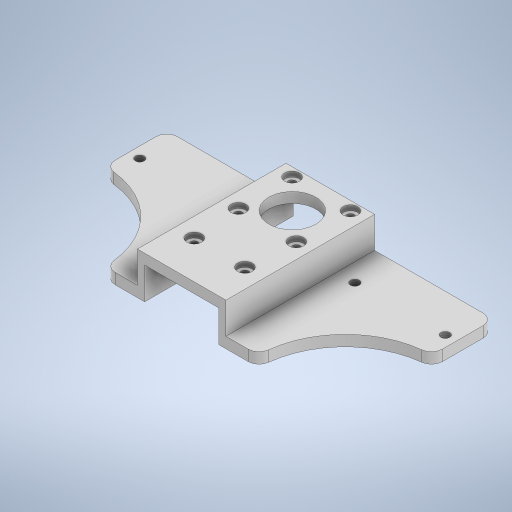
# Autodesk Inventor part: gripper_fixer
Saved by Autodesk Inventor 2024.2 (Build 282272000, 272)
## iProperties
Created: 2023-09-15
Part Number: gripper_fixer
Material: Generic
Document SubType Name: Modeling
Designer: 박동준
Density: 1 g/cm^3
Appearance: Default
Author: 박동준
Autodesk Inventor part; units mm, degrees
ref_plane "YZ Plane" through (0, 0, 0) normal (1, 0, 0) x (0, 1, 0)
ref_plane "XZ Plane" through (0, 0, 0) normal (0, 1, 0) x (-1, 0, 0)
ref_plane "XY Plane" through (0, 0, 0) normal (0, 0, 1) x (1, 0, 0)
sketch "Sketch1" plane through (0, 0, 0) normal (0, 0, 1) x (1, 0, 0)
  line L0 (-12.245, 11.65) -> (-12.245, 3)
  line L1 (-12.245, 3) -> (-45.245, 3)
  line L2 (-45.245, 3) -> (-45.245, 0)
  line L3 (-45.245, 0) -> (-10.245, 0)
  line L4 (-10.245, 0) -> (-10.245, 8.8)
  line L5 (-10.245, 8.8) -> (10.245, 8.8)
  line L6 (10.245, 8.8) -> (10.245, 0)
  line L7 (10.245, 0) -> (45.245, 0)
  line L8 (45.245, 0) -> (45.245, 3)
  line L9 (45.245, 3) -> (12.245, 3)
  line L10 (12.245, 3) -> (12.245, 11.65)
  line L11 (12.245, 11.65) -> (-12.245, 11.65)
  line L12 (-10.245, 0) -> (10.245, 0) construction
  point P0 (0, 0)
  point P1 (0, 11.65)
  point P2 (0, 0)
  point P3 (-12.245, 7.325)
  point P4 (12.245, 7.325)
  dimension "d0" = 20.49
  dimension "d1" = 2.85
  dimension "d3" = 5.8
  dimension "d4" = 3
  dimension "d5" = 3
  dimension "d6" = 35
  dimension "d7" = 35
  dimension "d73" = 33
  dimension "d74" = 33
  constraints: 26 end point, 9 perpendicular, 4 midpoint, 2 point on line, 2 vertical, 1 collinear, 1 horizontal alignment, 1 vertical alignment
  measures "d0" distance between parallel lines of L6 L4
  measures "d1" distance between parallel lines of L11 L5
  measures "d3" distance between parallel lines of L9 L5
  measures "d4" distance of L7.end L8.end
  measures "d5" distance of L1.end L2.end
  measures "d6" distance of L6.end L7.end
  measures "d7" distance of L2.end L3.end
  measures "d73" distance of L0.end L1.end
  measures "d74" distance of L8.end L9.end
extrude "Extrusion1" add sketch "Sketch1" along normal mid plane 41.1
sketch "Sketch8" plane through (12.245, 3, 20.55) normal (0, 1, 0) x (1, 0, 0)
  line L0 (0, 41.1) -> (0, 0)
  line L1 (33, 0) -> (0, 0) projected
  line L2 (33, 41.1) -> (33, 0) projected
  line L3 (0, 41.1) -> (33, 41.1) projected
  line L4 (-57.49, 41.1) -> (-57.49, 0) projected
  line L5 (-24.49, 0) -> (-57.49, 0) projected
  line L6 (-24.49, 0) -> (-24.49, 41.1) projected
  line L7 (-57.49, 41.1) -> (-24.49, 41.1) projected
  line L8 (33, 41.1) -> (33, 0) projected
  circle A0 centre (-11.645, 30.6) radius 6.4 projected
  line L9 (-12.245, 41) -> (-12.245, 0) construction
  point P0 (-12.245, 20.55)
  point P1 (-54.49, 30.65)
  point P2 (-29.49, 30.65)
  point P3 (-57.49, 20.55)
  point P4 (30, 30.65)
  point P5 (5, 30.65)
  dimension "d42" = 3
  dimension "d43" = 25
  dimension "d51" = 10.45
  dimension "d53" = 3
  constraints: 4 end point, 2 symmetric about line, 1 horizontal alignment, 1 midpoint, 1 vertical
  measures "d42" distance from line of L4 point (-54.49, 30.65)
  measures "d43" distance of point (-29.49, 30.65) point (-54.49, 30.65)
  measures "d51" distance from line of point (-29.49, 30.65) L7
  measures "d53" distance from line of L2 point (30, 30.65)
hole "Hole1" at (-42.245, 3, -10.1) at (-17.245, 3, -10.1) at (17.245, 3, -10.1) at (42.245, 3, -10.1) direction (0, -1, 0) diameter 2.459 end through all thread size "M3x0.5" class "6H" standard "ISO Metric profile"
sketch "Sketch9" plane through (12.245, 3, 20.55) normal (0, 1, 0) x (1, 0, 0)
  circle A0 centre (30, 30.65) radius 1.2295 projected
  circle A1 centre (5, 30.65) radius 1.2295 projected
  line L0 (0, 41.1) -> (0, 0) projected
  line L1 (33, 0) -> (0, 0) projected
  line L2 (33, 41.1) -> (33, 0) projected
  line L3 (0, 41.1) -> (33, 41.1) projected
  arc A2 (33, 24) -> (9, 0) centre (33, 0) ccw
  point P0 (-12.245, 20.55)
  dimension "d60" = 24
  constraints: 2 point on circle, 2 point on line, 1 centre point, 1 coincident
  measures "d60" radius of A2
extrude "Extrusion2" cut sketch "Sketch9" against normal blind 10 contours A2 L2 L1
mirror "Mirror1" about plane through (0, 0, 0) normal (1, 0, 0) of "Extrusion2"
sketch "Sketch10" plane through (-12.245, 11.65, 20.55) normal (0, 1, 0) x (1, 0, 0)
  circle A0 centre (12.245, 30.602) radius 6.5
  line L0 (0, 41.1) -> (0, 0) projected
  line L1 (24.49, 0) -> (0, 0) projected
  line L2 (24.49, 41.1) -> (24.49, 0) projected
  line L3 (0, 41.1) -> (24.49, 41.1) projected
  point P0 (12.245, 20.55)
  point P1 (12.245, 41.1)
  dimension "d75" = 13
  dimension "d76" = 10.498
  constraints: 1 centre point, 1 midpoint, 1 vertical alignment
  measures "d75" diameter of A0
  measures "d76" distance from line of L3 A0.centre
extrude "Extrusion3" cut sketch "Sketch10" against normal blind 10 contours A0
sketch "Sketch11" plane through (-12.245, 11.65, 20.55) normal (0, 1, 0) x (1, 0, 0)
  circle A0 centre (5.245, 10.482) radius 0.7835
  circle A1 centre (4.245, 23.702) radius 0.7835
  circle A2 centre (4.175, 38.602) radius 0.7835
  circle A3 centre (20.315, 38.602) radius 0.7835
  circle A4 centre (20.245, 23.702) radius 0.7835
  circle A5 centre (19.245, 10.482) radius 0.7835
  constraints: 6 centre point, 12 other
hole "Hole2" at (-8, 11.65, -3.152) at (8, 11.65, -3.152) at (8.07, 11.65, -18.052) at (-8.07, 11.65, -18.052) at (-7, 11.65, 10.068) at (7, 11.65, 10.068) direction (0, -1, 0) diameter 2.1 end through all counterbore diameter 4.1 counterbore depth 1.4
fillet "Fillet3" radius 3 6 edges at (-21.245, 1.5, 20.55) (-45.245, 1.5, -3.45) (-45.245, 1.5, -20.55) (21.245, 1.5, 20.55) (45.245, 1.5, -3.45) (45.245, 1.5, -20.55)
ref_plane "Work Plane1" through (0, 0, 0) normal (1, 0, 0) x (0, 1, 0)
body "Solid1"
